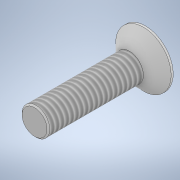
# Autodesk Inventor part: MM-MMount_to_Motor-CS_Bolt-
Saved by Autodesk Inventor 2020 (Build 240168000, 168)
## iProperties
Created: 2020-02-27
Part Number: MM-MMount_to_Motor-CS_Bolt-
Material: Generic
Document SubType Name: Modeling
Designer: Vitaliy
Density: 1 g/cm^3
Appearance: Default
Author: Vitaliy
Autodesk Inventor part; units mm, degrees
ref_plane "YZ Plane" through (0, 0, 0) normal (1, 0, 0) x (0, 1, 0)
ref_plane "XZ Plane" through (0, 0, 0) normal (0, 1, 0) x (-1, 0, 0)
ref_plane "XY Plane" through (0, 0, 0) normal (0, 0, 1) x (1, 0, 0)
sketch "Sketch1" plane through (0, 0, 0) normal (1, 0, 0) x (0, 1, 0)
  line L0 (0, 0) -> (0, -16)
  line L1 (0, -16) -> (4, -16)
  line L2 (2, 0) -> (0, 0)
  line L3 (2, 0) -> (2, -13.7)
  line L4 (2, -13.7) -> (4, -15.7)
  line L5 (4, -15.7) -> (4, -16)
  dimension "d0" = 16
  dimension "d4" = 2
  dimension "d5" = 2.3
  dimension "d6" = 45
  dimension "d7" = 4
  constraints: 12 end point, 2 vertical, 1 parallel, 1 perpendicular
  measures "d0" distance between parallel lines of L1 L2
  measures "d4" distance between parallel lines of L3 L0
  measures "d5" distance from line of L1 L3.end
  measures "d6" angle of L1 L4
  measures "d7" distance between parallel lines of L5 L0
revolve "Revolution1" add sketch "Sketch1" angle 360 about axis through (0, 0, 0) along (0, 0, -1)
sketch "Sketch2" plane through (0, 0, -16) normal (0, 0, -1) x (-1, 0, 0)
  line L0 (0, 1.4434) -> (1.25, 0.7217)
  line L1 (1.25, 0.7217) -> (1.25, -0.7217)
  line L2 (1.25, -0.7217) -> (0, -1.4434)
  line L3 (0, -1.4434) -> (-1.25, -0.7217)
  line L4 (-1.25, -0.7217) -> (-1.25, 0.7217)
  line L5 (-1.25, 0.7217) -> (0, 1.4434)
  point P0 (0, 0)
  point P1 (0, 0)
  dimension "d9" = 2.5
  constraints: 12 end point, 1 coincident, 13 other
  measures "d9" distance between parallel lines of L1 L4
extrude "Extrusion1" cut sketch "Sketch2" against normal blind 1.75
thread "Thread1" size "M4x0.7" class "6g" standard "ANSI Metric M Profile" length 24
chamfer "Chamfer1" distance 0.2 angle 45 1 edges at (0, -2, 0)
body "Solid1"
